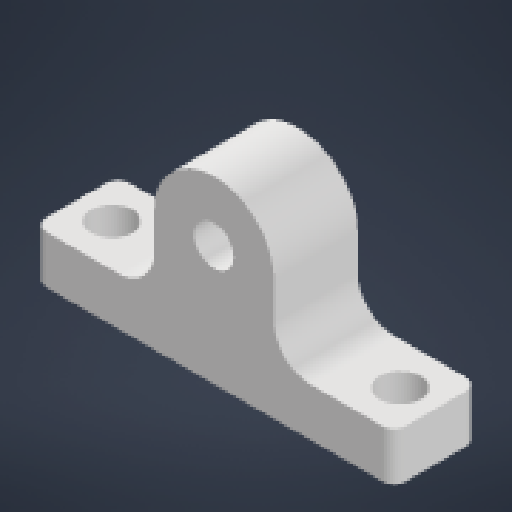
# Autodesk Inventor part: SoporteEjes
Saved by Autodesk Inventor 2026.3 (Build 303398000, 398)
## iProperties
Created: 2026-04-17
Part Number: SoporteEjes
Material: Genérico
Document SubType Name: Modeling
Designer: Jose Carlos
Density: 1 g/cm^3
Appearance: Valor por defecto
Author: Jose Carlos
Autodesk Inventor part; units mm, degrees
ref_plane "YZ Plane" through (0, 0, 0) normal (1, 0, 0) x (0, 1, 0)
ref_plane "XZ Plane" through (0, 0, 0) normal (0, 1, 0) x (-1, 0, 0)
ref_plane "XY Plane" through (0, 0, 0) normal (0, 0, 1) x (1, 0, 0)
sketch "Boceto1" plane through (0, 0, 0) normal (0, 0, 1) x (1, 0, 0)
  circle A0 centre (0, 0) radius 1.65
  line L0 (-15.5, -10) -> (35.5, -10) construction
  line L1 (5, -10) -> (-5, -10)
  line L2 (-5, -10) -> (-5, 5)
  line L3 (-5, 5) -> (5, 5)
  line L4 (5, 5) -> (5, -10)
  line L5 (-15, -10) -> (15, -10)
  line L6 (15, -10) -> (15, -6)
  line L7 (15, -6) -> (-15, -6)
  line L8 (-15, -6) -> (-15, -10)
  point P0 (-5, -6)
  point P1 (5, -6)
  dimension "d0" = 3.3
  dimension "d1" = 5
  dimension "d2" = 5
  dimension "d3" = 5
  dimension "d4" = 10
  dimension "d5" = 10
  dimension "d6" = 4
  constraints: 16 end point, 4 parallel, 2 horizontal, 2 perpendicular, 2 point on line, 1 centre point, 1 coincident
  measures "d0" diameter of A0
  measures "d1" distance from line of L4 point (0, 0)
  measures "d2" distance from line of L2 point (0, 0)
  measures "d3" distance from line of point (0, 0) L3
  measures "d4" distance between parallel lines of L2 L8
  measures "d5" distance between parallel lines of L4 L6
  measures "d6" distance of L7.end L5.start
extrude "Extrusión1" add sketch "Boceto1" along normal blind 1 and the other way blind 7 contours A0 | L1 L2 L7 L4 | L4 L7 L6 L5 | L5 L8 L7 L2 | L7 L2 L3 L4
sketch "Boceto2" plane through (-15, -6, -7) normal (0, 1, 0) x (-1, 0, 0)
  line L0 (-30, 0) -> (-20, 0) construction
  line L1 (-30, 0) -> (-30, 8) construction
  line L2 (0, 8) -> (-10, 8) construction
  line L3 (0, 0) -> (0, 8) construction
  line L4 (-20, 8) -> (-30, 8) projected
  point P0 (-15, 7)
  point P1 (-3, 3.5)
  point P2 (-27, 3.5)
  dimension "d35" = 3.5
  dimension "d36" = 3
  dimension "d37" = 3.5
  dimension "d38" = 3
  measures "d35" distance from line of L0 point (-27, 3.5)
  measures "d36" distance from line of L1 point (-27, 3.5)
  measures "d37" distance from line of L0 point (-3, 3.5)
  measures "d38" distance from line of L3 point (-3, 3.5)
hole "Agujero1" at (-12, -6, -3.5) at (12, -6, -3.5) direction (0, -1, 0) diameter 3.4 end through all
fillet "Empalme1" radius 5 2 edges at (-5, 5, -3) (5, 5, -3)
fillet "Empalme2" radius 3 2 edges at (-5, -6, -3) (5, -6, -3)
fillet "Empalme3" radius 1 4 edges at (-15, -8, -7) (-15, -8, 1) (15, -8, -7) (15, -8, 1)
sketch "Boceto6" plane through (0, 0, -7) normal (0, 0, -1) x (-1, 0, 0)
  point P0 (0, 0)
hole "Agujero3" at (0, 0, -7) direction (0, 0, 1) diameter 3.3 depth 7
